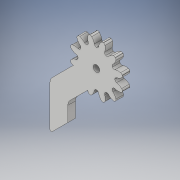
# Autodesk Inventor part: 齒輪2
Saved by Autodesk Inventor 2019 (Build 230136000, 136)
## iProperties
Created: 2022-01-10
Part Number: 齒輪2
Material: 一般
Document SubType Name: Modeling
Designer: 10617
Density: 1 g/cm^3
Appearance: 預設
Author: 10617
Autodesk Inventor part; units mm, degrees
ref_plane "YZ Plane" through (0, 0, 0) normal (1, 0, 0) x (0, 1, 0)
ref_plane "XZ Plane" through (0, 0, 0) normal (0, 1, 0) x (-1, 0, 0)
ref_plane "XY Plane" through (0, 0, 0) normal (0, 0, 1) x (1, 0, 0)
sketch "草圖1" plane through (0, 0, 0) normal (0, 0, 1) x (1, 0, 0)
  spline S0 degree 3 poles (12.8654, 17.3383) (12.6649, 17.124) (12.3633, 17.0366) (12.0794, 17.1107) knots 0 0 0 0 1 1 1 1
  line L0 (12.8654, 17.3383) -> (12.6649, 17.124) construction
  line L1 (12.6649, 17.124) -> (12.3633, 17.0366) construction
  line L2 (12.3633, 17.0366) -> (12.0794, 17.1107) construction
  spline S1 degree 3 poles (13.8808, 19.3219) (13.7347, 18.5786) (13.3829, 17.8913) (12.8654, 17.3383) knots 0 0 0 0 1 1 1 1
  line L3 (13.8808, 19.3219) -> (13.7347, 18.5786) construction
  line L4 (13.7347, 18.5786) -> (13.3829, 17.8913) construction
  line L5 (13.3829, 17.8913) -> (12.8654, 17.3383) construction
  spline S2 degree 3 poles (13.8808, 19.3219) (13.9607, 19.728) (14.3167, 20.021) (14.7306, 20.0211) knots 0 0 0 0 0.333333 0.333333 0.333333 0.333333
  line L6 (13.8808, 19.3219) -> (13.9607, 19.728) construction
  line L7 (13.9607, 19.728) -> (14.3167, 20.021) construction
  line L8 (14.3167, 20.021) -> (14.7306, 20.0211) construction
  spline S3 degree 3 poles (14.7306, 20.0211) (15.1446, 20.0212) (15.5009, 19.7285) (15.581, 19.3224) knots 0.333333 0.333333 0.333333 0.333333 1 1 1 1
  line L9 (14.7306, 20.0211) -> (15.1446, 20.0212) construction
  line L10 (15.1446, 20.0212) -> (15.5009, 19.7285) construction
  line L11 (15.5009, 19.7285) -> (15.581, 19.3224) construction
  spline S4 degree 3 poles (16.5979, 17.3395) (16.08, 17.8923) (15.7277, 18.5793) (15.581, 19.3224) knots 0 0 0 0 1 1 1 1
  line L12 (16.5979, 17.3395) -> (16.08, 17.8923) construction
  line L13 (16.08, 17.8923) -> (15.7277, 18.5793) construction
  line L14 (15.7277, 18.5793) -> (15.581, 19.3224) construction
  spline S5 degree 3 poles (17.384, 17.1126) (17.1002, 17.0383) (16.7985, 17.1254) (16.5979, 17.3395) knots 0 0 0 0 1 1 1 1
  line L15 (17.384, 17.1126) -> (17.1002, 17.0383) construction
  line L16 (17.1002, 17.0383) -> (16.7985, 17.1254) construction
  line L17 (16.7985, 17.1254) -> (16.5979, 17.3395) construction
  spline S6 degree 3 poles (17.5145, 17.1475) (17.4711, 17.1356) (17.4276, 17.1239) (17.384, 17.1126) knots 0 0 0 0 1 1 1 1
  line L18 (17.5145, 17.1475) -> (17.4711, 17.1356) construction
  line L19 (17.4711, 17.1356) -> (17.4276, 17.1239) construction
  line L20 (17.4276, 17.1239) -> (17.384, 17.1126) construction
  spline S7 degree 3 poles (18.0814, 17.7376) (18.0149, 17.4518) (17.7973, 17.2254) (17.5145, 17.1475) knots 0 0 0 0 1 1 1 1
  line L21 (18.0814, 17.7376) -> (18.0149, 17.4518) construction
  line L22 (18.0149, 17.4518) -> (17.7973, 17.2254) construction
  line L23 (17.7973, 17.2254) -> (17.5145, 17.1475) construction
  spline S8 degree 3 poles (17.969, 19.9632) (18.214, 19.2465) (18.253, 18.4754) (18.0814, 17.7376) knots 0 0 0 0 1 1 1 1
  line L24 (17.969, 19.9632) -> (18.214, 19.2465) construction
  line L25 (18.214, 19.2465) -> (18.253, 18.4754) construction
  line L26 (18.253, 18.4754) -> (18.0814, 17.7376) construction
  spline S9 degree 3 poles (18.3553, 20.9937) (18.7138, 21.2008) (19.1686, 21.1254) (19.4411, 20.8138) knots 0.333333 0.333333 0.333333 0.333333 1 1 1 1
  line L27 (18.3553, 20.9937) -> (18.7138, 21.2008) construction
  line L28 (18.7138, 21.2008) -> (19.1686, 21.1254) construction
  line L29 (19.1686, 21.1254) -> (19.4411, 20.8138) construction
  spline S10 degree 3 poles (21.3132, 19.605) (20.5884, 19.8247) (19.9397, 20.2436) (19.4411, 20.8138) knots 0 0 0 0 1 1 1 1
  line L30 (21.3132, 19.605) -> (20.5884, 19.8247) construction
  line L31 (20.5884, 19.8247) -> (19.9397, 20.2436) construction
  line L32 (19.9397, 20.2436) -> (19.4411, 20.8138) construction
  spline S11 degree 3 poles (22.1075, 19.8015) (21.8988, 19.5953) (21.594, 19.5199) (21.3132, 19.605) knots 0 0 0 0 1 1 1 1
  line L33 (22.1075, 19.8015) -> (21.8988, 19.5953) construction
  line L34 (21.8988, 19.5953) -> (21.594, 19.5199) construction
  line L35 (21.594, 19.5199) -> (21.3132, 19.605) construction
  spline S12 degree 3 poles (22.203, 19.897) (22.1713, 19.8649) (22.1395, 19.8331) (22.1075, 19.8015) knots 0 0 0 0 1 1 1 1
  line L36 (22.203, 19.897) -> (22.1713, 19.8649) construction
  line L37 (22.1713, 19.8649) -> (22.1395, 19.8331) construction
  line L38 (22.1395, 19.8331) -> (22.1075, 19.8015) construction
  spline S13 degree 3 poles (22.3988, 20.6914) (22.4841, 20.4107) (22.409, 20.1059) (22.203, 19.897) knots 0 0 0 0 1 1 1 1
  line L39 (22.3988, 20.6914) -> (22.4841, 20.4107) construction
  line L40 (22.4841, 20.4107) -> (22.409, 20.1059) construction
  line L41 (22.409, 20.1059) -> (22.203, 19.897) construction
  spline S14 degree 3 poles (21.1888, 22.5627) (20.8769, 22.8349) (20.8012, 23.2897) (21.0082, 23.6484) knots 0 0 0 0 0.333333 0.333333 0.333333 0.333333
  line L42 (21.1888, 22.5627) -> (20.8769, 22.8349) construction
  line L43 (20.8769, 22.8349) -> (20.8012, 23.2897) construction
  line L44 (20.8012, 23.2897) -> (21.0082, 23.6484) construction
  spline S15 degree 3 poles (21.1888, 22.5627) (21.7593, 22.0645) (22.1786, 21.4162) (22.3988, 20.6914) knots 0 0 0 0 1 1 1 1
  line L45 (21.1888, 22.5627) -> (21.7593, 22.0645) construction
  line L46 (21.7593, 22.0645) -> (22.1786, 21.4162) construction
  line L47 (22.1786, 21.4162) -> (22.3988, 20.6914) construction
  spline S16 degree 3 poles (21.0082, 23.6484) (21.215, 24.0069) (21.6465, 24.1691) (22.0384, 24.0354) knots 0.333333 0.333333 0.333333 0.333333 1 1 1 1
  line L48 (21.0082, 23.6484) -> (21.215, 24.0069) construction
  line L49 (21.215, 24.0069) -> (21.6465, 24.1691) construction
  line L50 (21.6465, 24.1691) -> (22.0384, 24.0354) construction
  spline S17 degree 3 poles (24.264, 23.9245) (23.5264, 23.7525) (22.7552, 23.7908) (22.0384, 24.0354) knots 0 0 0 0 1 1 1 1
  line L51 (24.264, 23.9245) -> (23.5264, 23.7525) construction
  line L52 (23.5264, 23.7525) -> (22.7552, 23.7908) construction
  line L53 (22.7552, 23.7908) -> (22.0384, 24.0354) construction
  spline S18 degree 3 poles (24.8536, 24.4919) (24.776, 24.209) (24.5497, 23.9912) (24.264, 23.9245) knots 0 0 0 0 1 1 1 1
  line L54 (24.8536, 24.4919) -> (24.776, 24.209) construction
  line L55 (24.776, 24.209) -> (24.5497, 23.9912) construction
  line L56 (24.5497, 23.9912) -> (24.264, 23.9245) construction
  spline S19 degree 3 poles (24.8885, 24.6223) (24.8772, 24.5788) (24.8656, 24.5353) (24.8536, 24.4919) knots 0 0 0 0 1 1 1 1
  line L57 (24.8885, 24.6223) -> (24.8772, 24.5788) construction
  line L58 (24.8772, 24.5788) -> (24.8656, 24.5353) construction
  line L59 (24.8656, 24.5353) -> (24.8536, 24.4919) construction
  spline S20 degree 3 poles (24.6611, 25.4083) (24.8753, 25.2078) (24.9626, 24.9062) (24.8885, 24.6223) knots 0 0 0 0 1 1 1 1
  line L60 (24.6611, 25.4083) -> (24.8753, 25.2078) construction
  line L61 (24.8753, 25.2078) -> (24.9626, 24.9062) construction
  line L62 (24.9626, 24.9062) -> (24.8885, 24.6223) construction
  spline S21 degree 3 poles (17.969, 19.9632) (17.835, 20.3549) (17.997, 20.7866) (18.3553, 20.9937) knots 0 0 0 0 0.333333 0.333333 0.333333 0.333333
  line L63 (17.969, 19.9632) -> (17.835, 20.3549) construction
  line L64 (17.835, 20.3549) -> (17.997, 20.7866) construction
  line L65 (17.997, 20.7866) -> (18.3553, 20.9937) construction
  spline S22 degree 3 poles (22.6775, 26.4238) (23.4206, 26.2777) (24.1079, 25.9258) (24.6611, 25.4083) knots 0 0 0 0 1 1 1 1
  line L66 (22.6775, 26.4238) -> (23.4206, 26.2777) construction
  line L67 (23.4206, 26.2777) -> (24.1079, 25.9258) construction
  line L68 (24.1079, 25.9258) -> (24.6611, 25.4083) construction
  spline S23 degree 3 poles (22.6775, 26.4238) (22.2712, 26.5037) (21.9783, 26.8597) (21.9782, 27.2738) knots 0 0 0 0 0.333333 0.333333 0.333333 0.333333
  line L69 (22.6775, 26.4238) -> (22.2712, 26.5037) construction
  line L70 (22.2712, 26.5037) -> (21.9783, 26.8597) construction
  line L71 (21.9783, 26.8597) -> (21.9782, 27.2738) construction
  spline S24 degree 3 poles (24.6597, 29.1408) (24.107, 28.6229) (23.4199, 28.2706) (22.6768, 28.124) knots 0 0 0 0 1 1 1 1
  line L72 (24.6597, 29.1408) -> (24.107, 28.6229) construction
  line L73 (24.107, 28.6229) -> (23.4199, 28.2706) construction
  line L74 (23.4199, 28.2706) -> (22.6768, 28.124) construction
  spline S25 degree 3 poles (22.036, 30.512) (21.6444, 30.3781) (21.2127, 30.5399) (21.0056, 30.8983) knots 0 0 0 0 0.333333 0.333333 0.333333 0.333333
  line L75 (22.036, 30.512) -> (21.6444, 30.3781) construction
  line L76 (21.6444, 30.3781) -> (21.2127, 30.5399) construction
  line L77 (21.2127, 30.5399) -> (21.0056, 30.8983) construction
  spline S26 degree 3 poles (24.8868, 29.927) (24.9609, 29.6432) (24.8738, 29.3414) (24.6597, 29.1408) knots 0 0 0 0 1 1 1 1
  line L78 (24.8868, 29.927) -> (24.9609, 29.6432) construction
  line L79 (24.9609, 29.6432) -> (24.8738, 29.3414) construction
  line L80 (24.8738, 29.3414) -> (24.6597, 29.1408) construction
  spline S27 degree 3 poles (24.8517, 30.0574) (24.8637, 30.014) (24.8753, 29.9705) (24.8868, 29.927) knots 0 0 0 0 1 1 1 1
  line L81 (24.8517, 30.0574) -> (24.8637, 30.014) construction
  line L82 (24.8637, 30.014) -> (24.8753, 29.9705) construction
  line L83 (24.8753, 29.9705) -> (24.8868, 29.927) construction
  spline S28 degree 3 poles (22.036, 30.512) (22.7528, 30.7571) (23.5239, 30.796) (24.2617, 30.6243) knots 0 0 0 0 1 1 1 1
  line L84 (22.036, 30.512) -> (22.7528, 30.7571) construction
  line L85 (22.7528, 30.7571) -> (23.5239, 30.796) construction
  line L86 (23.5239, 30.796) -> (24.2617, 30.6243) construction
  spline S29 degree 3 poles (24.2617, 30.6243) (24.5474, 30.5578) (24.7738, 30.3403) (24.8517, 30.0574) knots 0 0 0 0 1 1 1 1
  line L87 (24.2617, 30.6243) -> (24.5474, 30.5578) construction
  line L88 (24.5474, 30.5578) -> (24.7738, 30.3403) construction
  line L89 (24.7738, 30.3403) -> (24.8517, 30.0574) construction
  spline S30 degree 3 poles (21.0056, 30.8983) (20.7984, 31.2568) (20.8738, 31.7116) (21.1855, 31.984) knots 0.333333 0.333333 0.333333 0.333333 1 1 1 1
  line L90 (21.0056, 30.8983) -> (20.7984, 31.2568) construction
  line L91 (20.7984, 31.2568) -> (20.8738, 31.7116) construction
  line L92 (20.8738, 31.7116) -> (21.1855, 31.984) construction
  spline S31 degree 3 poles (19.4365, 33.7317) (19.1643, 33.4199) (18.7095, 33.3442) (18.3509, 33.5511) knots 0 0 0 0 0.333333 0.333333 0.333333 0.333333
  line L93 (19.4365, 33.7317) -> (19.1643, 33.4199) construction
  line L94 (19.1643, 33.4199) -> (18.7095, 33.3442) construction
  line L95 (18.7095, 33.3442) -> (18.3509, 33.5511) construction
  spline S32 degree 3 poles (22.3942, 33.8562) (22.1745, 33.1313) (21.7557, 32.4826) (21.1855, 31.984) knots 0 0 0 0 1 1 1 1
  line L96 (22.3942, 33.8562) -> (22.1745, 33.1313) construction
  line L97 (22.1745, 33.1313) -> (21.7557, 32.4826) construction
  line L98 (21.7557, 32.4826) -> (21.1855, 31.984) construction
  spline S33 degree 3 poles (22.1022, 34.7459) (22.1343, 34.7143) (22.1661, 34.6825) (22.1978, 34.6504) knots 0 0 0 0 1 1 1 1
  line L99 (22.1022, 34.7459) -> (22.1343, 34.7143) construction
  line L100 (22.1343, 34.7143) -> (22.1661, 34.6825) construction
  line L101 (22.1661, 34.6825) -> (22.1978, 34.6504) construction
  spline S34 degree 3 poles (22.1978, 34.6504) (22.404, 34.4418) (22.4793, 34.1369) (22.3942, 33.8562) knots 0 0 0 0 1 1 1 1
  line L102 (22.1978, 34.6504) -> (22.404, 34.4418) construction
  line L103 (22.404, 34.4418) -> (22.4793, 34.1369) construction
  line L104 (22.4793, 34.1369) -> (22.3942, 33.8562) construction
  spline S35 degree 3 poles (19.4365, 33.7317) (19.9347, 34.3023) (20.583, 34.7216) (21.3078, 34.9419) knots 0 0 0 0 1 1 1 1
  line L105 (19.4365, 33.7317) -> (19.9347, 34.3023) construction
  line L106 (19.9347, 34.3023) -> (20.583, 34.7216) construction
  line L107 (20.583, 34.7216) -> (21.3078, 34.9419) construction
  spline S36 degree 3 poles (21.3078, 34.9419) (21.5885, 35.0272) (21.8933, 34.952) (22.1022, 34.7459) knots 0 0 0 0 1 1 1 1
  line L108 (21.3078, 34.9419) -> (21.5885, 35.0272) construction
  line L109 (21.5885, 35.0272) -> (21.8933, 34.952) construction
  line L110 (21.8933, 34.952) -> (22.1022, 34.7459) construction
  spline S37 degree 3 poles (21.9782, 27.2738) (21.978, 27.6877) (22.2707, 28.0438) (22.6768, 28.124) knots 0.333333 0.333333 0.333333 0.333333 1 1 1 1
  line L111 (21.9782, 27.2738) -> (21.978, 27.6877) construction
  line L112 (21.978, 27.6877) -> (22.2707, 28.0438) construction
  line L113 (22.2707, 28.0438) -> (22.6768, 28.124) construction
  spline S38 degree 3 poles (18.3509, 33.5511) (17.9924, 33.7579) (17.8301, 34.1895) (17.9638, 34.5813) knots 0.333333 0.333333 0.333333 0.333333 1 1 1 1
  line L114 (18.3509, 33.5511) -> (17.9924, 33.7579) construction
  line L115 (17.9924, 33.7579) -> (17.8301, 34.1895) construction
  line L116 (17.8301, 34.1895) -> (17.9638, 34.5813) construction
  spline S39 degree 3 poles (18.0747, 36.8069) (18.2468, 36.0694) (18.2084, 35.2982) (17.9638, 34.5813) knots 0 0 0 0 1 1 1 1
  line L117 (18.0747, 36.8069) -> (18.2468, 36.0694) construction
  line L118 (18.2468, 36.0694) -> (18.2084, 35.2982) construction
  line L119 (18.2084, 35.2982) -> (17.9638, 34.5813) construction
  spline S40 degree 3 poles (17.5073, 37.3967) (17.7903, 37.3189) (18.008, 37.0927) (18.0747, 36.8069) knots 0 0 0 0 1 1 1 1
  line L120 (17.5073, 37.3967) -> (17.7903, 37.3189) construction
  line L121 (17.7903, 37.3189) -> (18.008, 37.0927) construction
  line L122 (18.008, 37.0927) -> (18.0747, 36.8069) construction
  spline S41 degree 3 poles (15.5755, 35.2204) (15.4955, 34.8142) (15.1395, 34.5212) (14.7255, 34.5211) knots 0 0 0 0 0.333333 0.333333 0.333333 0.333333
  line L123 (15.5755, 35.2204) -> (15.4955, 34.8142) construction
  line L124 (15.4955, 34.8142) -> (15.1395, 34.5212) construction
  line L125 (15.1395, 34.5212) -> (14.7255, 34.5211) construction
  spline S42 degree 3 poles (17.3769, 37.4315) (17.4205, 37.4202) (17.4639, 37.4085) (17.5073, 37.3967) knots 0 0 0 0 1 1 1 1
  line L126 (17.3769, 37.4315) -> (17.4205, 37.4202) construction
  line L127 (17.4205, 37.4202) -> (17.4639, 37.4085) construction
  line L128 (17.4639, 37.4085) -> (17.5073, 37.3967) construction
  spline S43 degree 3 poles (16.591, 37.204) (16.7914, 37.4182) (17.093, 37.5055) (17.3769, 37.4315) knots 0 0 0 0 1 1 1 1
  line L129 (16.591, 37.204) -> (16.7914, 37.4182) construction
  line L130 (16.7914, 37.4182) -> (17.093, 37.5055) construction
  line L131 (17.093, 37.5055) -> (17.3769, 37.4315) construction
  spline S44 degree 3 poles (15.5755, 35.2204) (15.7216, 35.9636) (16.0734, 36.6508) (16.591, 37.204) knots 0 0 0 0 1 1 1 1
  line L132 (15.5755, 35.2204) -> (15.7216, 35.9636) construction
  line L133 (15.7216, 35.9636) -> (16.0734, 36.6508) construction
  line L134 (16.0734, 36.6508) -> (16.591, 37.204) construction
  spline S45 degree 3 poles (14.7255, 34.5211) (14.3116, 34.5209) (13.9554, 34.8136) (13.8752, 35.2198) knots 0.333333 0.333333 0.333333 0.333333 1 1 1 1
  line L135 (14.7255, 34.5211) -> (14.3116, 34.5209) construction
  line L136 (14.3116, 34.5209) -> (13.9554, 34.8136) construction
  line L137 (13.9554, 34.8136) -> (13.8752, 35.2198) construction
  spline S46 degree 3 poles (11.4873, 34.5791) (11.6211, 34.1873) (11.4593, 33.7556) (11.101, 33.5485) knots 0 0 0 0 0.333333 0.333333 0.333333 0.333333
  line L138 (11.4873, 34.5791) -> (11.6211, 34.1873) construction
  line L139 (11.6211, 34.1873) -> (11.4593, 33.7556) construction
  line L140 (11.4593, 33.7556) -> (11.101, 33.5485) construction
  spline S47 degree 3 poles (12.0723, 37.4297) (12.356, 37.5039) (12.6578, 37.4167) (12.8584, 37.2026) knots 0 0 0 0 1 1 1 1
  line L141 (12.0723, 37.4297) -> (12.356, 37.5039) construction
  line L142 (12.356, 37.5039) -> (12.6578, 37.4167) construction
  line L143 (12.6578, 37.4167) -> (12.8584, 37.2026) construction
  spline S48 degree 3 poles (11.4873, 34.5791) (11.2423, 35.2957) (11.2033, 36.0668) (11.375, 36.8046) knots 0 0 0 0 1 1 1 1
  line L144 (11.4873, 34.5791) -> (11.2423, 35.2957) construction
  line L145 (11.2423, 35.2957) -> (11.2033, 36.0668) construction
  line L146 (11.2033, 36.0668) -> (11.375, 36.8046) construction
  spline S49 degree 3 poles (11.9418, 37.3947) (11.9852, 37.4066) (12.0287, 37.4183) (12.0723, 37.4297) knots 0 0 0 0 1 1 1 1
  line L147 (11.9418, 37.3947) -> (11.9852, 37.4066) construction
  line L148 (11.9852, 37.4066) -> (12.0287, 37.4183) construction
  line L149 (12.0287, 37.4183) -> (12.0723, 37.4297) construction
  spline S50 degree 3 poles (11.375, 36.8046) (11.4414, 37.0903) (11.659, 37.3168) (11.9418, 37.3947) knots 0 0 0 0 1 1 1 1
  line L150 (11.375, 36.8046) -> (11.4414, 37.0903) construction
  line L151 (11.4414, 37.0903) -> (11.659, 37.3168) construction
  line L152 (11.659, 37.3168) -> (11.9418, 37.3947) construction
  spline S51 degree 3 poles (12.8584, 37.2026) (13.3763, 36.6499) (13.7286, 35.9629) (13.8752, 35.2198) knots 0 0 0 0 1 1 1 1
  line L153 (12.8584, 37.2026) -> (13.3763, 36.6499) construction
  line L154 (13.3763, 36.6499) -> (13.7286, 35.9629) construction
  line L155 (13.7286, 35.9629) -> (13.8752, 35.2198) construction
  spline S52 degree 3 poles (4.5696, 24.6152) (4.4954, 24.8991) (4.5825, 25.2007) (4.7966, 25.4013) knots 0 0 0 0 1 1 1 1
  line L156 (4.5696, 24.6152) -> (4.4954, 24.8991) construction
  line L157 (4.4954, 24.8991) -> (4.5825, 25.2007) construction
  line L158 (4.5825, 25.2007) -> (4.7966, 25.4013) construction
  spline S53 degree 3 poles (4.6046, 24.4847) (4.5926, 24.5282) (4.581, 24.5717) (4.5696, 24.6152) knots 0 0 0 0 1 1 1 1
  line L159 (4.6046, 24.4847) -> (4.5926, 24.5282) construction
  line L160 (4.5926, 24.5282) -> (4.581, 24.5717) construction
  line L161 (4.581, 24.5717) -> (4.5696, 24.6152) construction
  spline S54 degree 3 poles (5.1946, 23.9179) (4.9089, 23.9844) (4.6825, 24.2019) (4.6046, 24.4847) knots 0 0 0 0 1 1 1 1
  line L162 (5.1946, 23.9179) -> (4.9089, 23.9844) construction
  line L163 (4.9089, 23.9844) -> (4.6825, 24.2019) construction
  line L164 (4.6825, 24.2019) -> (4.6046, 24.4847) construction
  spline S55 degree 3 poles (5.6443, 23.8397) (5.493, 23.8573) (5.3429, 23.8834) (5.1946, 23.9179) knots 0 0 0 0 1 1 1 1
  line L165 (5.6443, 23.8397) -> (5.493, 23.8573) construction
  line L166 (5.493, 23.8573) -> (5.3429, 23.8834) construction
  line L167 (5.3429, 23.8834) -> (5.1946, 23.9179) construction
  spline S56 degree 3 poles (11.101, 33.5485) (10.7425, 33.3414) (10.2877, 33.4168) (10.0152, 33.7285) knots 0.333333 0.333333 0.333333 0.333333 1 1 1 1
  line L168 (11.101, 33.5485) -> (10.7425, 33.3414) construction
  line L169 (10.7425, 33.3414) -> (10.2877, 33.4168) construction
  line L170 (10.2877, 33.4168) -> (10.0152, 33.7285) construction
  circle A0 centre (14.7281, 27.2712) radius 1.3
  spline S57 degree 3 poles (8.1431, 34.9373) (8.8679, 34.7175) (9.5166, 34.2987) (10.0152, 33.7285) knots 0 0 0 0 1 1 1 1
  line L171 (8.1431, 34.9373) -> (8.8679, 34.7175) construction
  line L172 (8.8679, 34.7175) -> (9.5166, 34.2987) construction
  line L173 (9.5166, 34.2987) -> (10.0152, 33.7285) construction
  spline S58 degree 3 poles (7.3488, 34.7408) (7.5575, 34.9469) (7.8623, 35.0223) (8.1431, 34.9373) knots 0 0 0 0 1 1 1 1
  line L174 (7.3488, 34.7408) -> (7.5575, 34.9469) construction
  line L175 (7.5575, 34.9469) -> (7.8623, 35.0223) construction
  line L176 (7.8623, 35.0223) -> (8.1431, 34.9373) construction
  spline S59 degree 3 poles (7.2533, 34.6452) (7.285, 34.6772) (7.3168, 34.7091) (7.3488, 34.7408) knots 0 0 0 0 1 1 1 1
  line L177 (7.2533, 34.6452) -> (7.285, 34.6772) construction
  line L178 (7.285, 34.6772) -> (7.3168, 34.7091) construction
  line L179 (7.3168, 34.7091) -> (7.3488, 34.7408) construction
  spline S60 degree 3 poles (7.0575, 33.8508) (6.9721, 34.1316) (7.0473, 34.4364) (7.2533, 34.6452) knots 0 0 0 0 1 1 1 1
  line L180 (7.0575, 33.8508) -> (6.9721, 34.1316) construction
  line L181 (6.9721, 34.1316) -> (7.0473, 34.4364) construction
  line L182 (7.0473, 34.4364) -> (7.2533, 34.6452) construction
  spline S61 degree 3 poles (8.2676, 31.9796) (7.697, 32.4777) (7.2777, 33.1261) (7.0575, 33.8508) knots 0 0 0 0 1 1 1 1
  line L183 (8.2676, 31.9796) -> (7.697, 32.4777) construction
  line L184 (7.697, 32.4777) -> (7.2777, 33.1261) construction
  line L185 (7.2777, 33.1261) -> (7.0575, 33.8508) construction
  spline S62 degree 3 poles (8.4482, 30.894) (8.2413, 30.5353) (7.8098, 30.3732) (7.418, 30.5068) knots 0.333333 0.333333 0.333333 0.333333 1 1 1 1
  line L186 (8.4482, 30.894) -> (8.2413, 30.5353) construction
  line L187 (8.2413, 30.5353) -> (7.8098, 30.3732) construction
  line L188 (7.8098, 30.3732) -> (7.418, 30.5068) construction
  spline S63 degree 3 poles (5.1923, 30.6176) (5.9299, 30.7897) (6.7011, 30.7514) (7.418, 30.5068) knots 0 0 0 0 1 1 1 1
  line L189 (5.1923, 30.6176) -> (5.9299, 30.7897) construction
  line L190 (5.9299, 30.7897) -> (6.7011, 30.7514) construction
  line L191 (6.7011, 30.7514) -> (7.418, 30.5068) construction
  spline S64 degree 3 poles (6.7788, 28.1184) (7.1851, 28.0386) (7.478, 27.6825) (7.4782, 27.2686) knots 0 0 0 0 0.333333 0.333333 0.333333 0.333333
  line L192 (6.7788, 28.1184) -> (7.1851, 28.0386) construction
  line L193 (7.1851, 28.0386) -> (7.478, 27.6825) construction
  line L194 (7.478, 27.6825) -> (7.4782, 27.2686) construction
  spline S65 degree 3 poles (7.4782, 27.2686) (7.4783, 26.8546) (7.1856, 26.4984) (6.7795, 26.4183) knots 0.333333 0.333333 0.333333 0.333333 1 1 1 1
  line L195 (7.4782, 27.2686) -> (7.4783, 26.8546) construction
  line L196 (7.4783, 26.8546) -> (7.1856, 26.4984) construction
  line L197 (7.1856, 26.4984) -> (6.7795, 26.4183) construction
  spline S66 degree 3 poles (4.6027, 30.0503) (4.6803, 30.3332) (4.9065, 30.551) (5.1923, 30.6176) knots 0 0 0 0 1 1 1 1
  line L198 (4.6027, 30.0503) -> (4.6803, 30.3332) construction
  line L199 (4.6803, 30.3332) -> (4.9065, 30.551) construction
  line L200 (4.9065, 30.551) -> (5.1923, 30.6176) construction
  spline S67 degree 3 poles (4.5677, 29.9198) (4.5791, 29.9634) (4.5907, 30.007) (4.6027, 30.0503) knots 0 0 0 0 1 1 1 1
  line L201 (4.5677, 29.9198) -> (4.5791, 29.9634) construction
  line L202 (4.5791, 29.9634) -> (4.5907, 30.007) construction
  line L203 (4.5907, 30.007) -> (4.6027, 30.0503) construction
  spline S68 degree 3 poles (4.7952, 29.1339) (4.581, 29.3343) (4.4937, 29.636) (4.5677, 29.9198) knots 0 0 0 0 1 1 1 1
  line L204 (4.7952, 29.1339) -> (4.581, 29.3343) construction
  line L205 (4.581, 29.3343) -> (4.4937, 29.636) construction
  line L206 (4.4937, 29.636) -> (4.5677, 29.9198) construction
  spline S69 degree 3 poles (6.7788, 28.1184) (6.0357, 28.2645) (5.3484, 28.6163) (4.7952, 29.1339) knots 0 0 0 0 1 1 1 1
  line L207 (6.7788, 28.1184) -> (6.0357, 28.2645) construction
  line L208 (6.0357, 28.2645) -> (5.3484, 28.6163) construction
  line L209 (5.3484, 28.6163) -> (4.7952, 29.1339) construction
  spline S70 degree 3 poles (4.7966, 25.4013) (5.3493, 25.9192) (6.0363, 26.2715) (6.7795, 26.4183) knots 0 0 0 0 1 1 1 1
  line L210 (4.7966, 25.4013) -> (5.3493, 25.9192) construction
  line L211 (5.3493, 25.9192) -> (6.0363, 26.2715) construction
  line L212 (6.0363, 26.2715) -> (6.7795, 26.4183) construction
  spline S71 degree 3 poles (8.2676, 31.9796) (8.5794, 31.7073) (8.655, 31.2524) (8.4482, 30.894) knots 0 0 0 0 0.333333 0.333333 0.333333 0.333333
  line L213 (8.2676, 31.9796) -> (8.5794, 31.7073) construction
  line L214 (8.5794, 31.7073) -> (8.655, 31.2524) construction
  line L215 (8.655, 31.2524) -> (8.4482, 30.894) construction
  arc A1 (-2.7385, 15.4511) -> (-3.6164, 13.3294) centre (-0.6164, 13.3306) ccw
  spline S72 degree 3 poles (12.0794, 17.1107) (12.0358, 17.122) (11.9924, 17.1337) (11.9489, 17.1456) knots 0 0 0 0 1 1 1 1
  line L216 (12.0794, 17.1107) -> (12.0358, 17.122) construction
  line L217 (12.0358, 17.122) -> (11.9924, 17.1337) construction
  line L218 (11.9924, 17.1337) -> (11.9489, 17.1456) construction
  spline S73 degree 3 poles (11.3816, 17.7352) (11.347, 17.8835) (11.3208, 18.0336) (11.3031, 18.1849) knots 0 0 0 0 1 1 1 1
  line L219 (11.3816, 17.7352) -> (11.347, 17.8835) construction
  line L220 (11.347, 17.8835) -> (11.3208, 18.0336) construction
  line L221 (11.3208, 18.0336) -> (11.3031, 18.1849) construction
  line L222 (5.6443, 23.8397) -> (-2.7385, 15.4511)
  line L223 (4.3341, 11.211) -> (11.3031, 18.1849)
  arc A2 (4.3341, 11.211) -> (3.4562, 9.0893) centre (6.4558, 9.0906) ccw
  line L224 (3.4562, 9.0893) -> (3.4582, 3.1902)
  line L225 (-3.6164, 13.3294) -> (-3.6163, 3.8294)
  line L226 (3.4582, 3.1902) -> (-2.7582, -3.0307)
  line L227 (-3.6107, -2.6763) -> (-3.6163, 3.8294)
  arc A3 (-3.6107, -2.6763) -> (-2.7582, -3.0307) centre (-3.1107, -2.6761) ccw
  spline S74 degree 3 poles (11.9489, 17.1456) (11.666, 17.2232) (11.4483, 17.4496) (11.3816, 17.7352) knots 0 0 0 0 1 1 1 1
  line L228 (11.9489, 17.1456) -> (11.666, 17.2232) construction
  line L229 (11.666, 17.2232) -> (11.4483, 17.4496) construction
  line L230 (11.4483, 17.4496) -> (11.3816, 17.7352) construction
  point P0 (0, 0)
  constraints: 12 end point, 6 point on circle, 4 centre point, 225 other
extrude "擠出1" add sketch "草圖1" along normal blind 3
